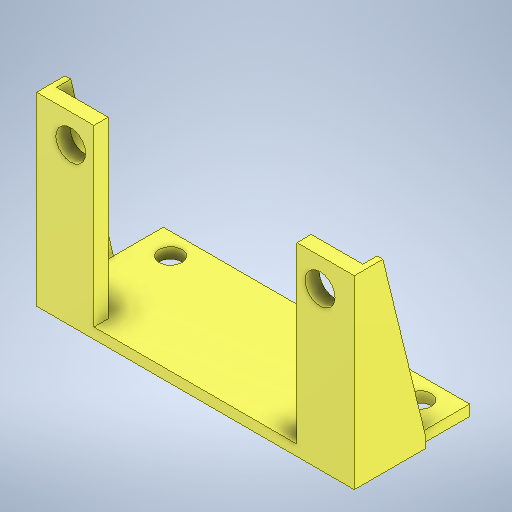
# Autodesk Inventor part: 28BYJ-48_Braket3
Saved by Autodesk Inventor 2025.3 (Build 293356030, 356C)
## iProperties
Created: 2025-07-13
Part Number: 28BYJ-48_Braket3
Material: 一般
Document SubType Name: Modeling
Designer: daisuke
Density: 1 g/cm^3
Appearance: 滑らか - 黄
Author: daisuke
Autodesk Inventor part; units mm, degrees
ref_plane "YZ Plane" through (0, 0, 0) normal (1, 0, 0) x (0, 1, 0)
ref_plane "XZ Plane" through (0, 0, 0) normal (0, 1, 0) x (-1, 0, 0)
ref_plane "XY Plane" through (0, 0, 0) normal (0, 0, 1) x (1, 0, 0)
sketch "スケッチ1" plane through (0, 0, 0) normal (0, 0, 1) x (1, 0, 0)
  line L0 (0, 0) -> (0, 23.3181) construction
  line L1 (-22.6457, 22) -> (22.6457, 22) construction
  line L2 (-20.3832, 1.5) -> (20.3832, 1.5) construction
  circle A0 centre (0, 22) radius 14 construction
  line L3 (-22.6457, 14) -> (22.6457, 14) construction
  circle A1 centre (-17.5, 22) radius 2.1
  circle A2 centre (17.5, 22) radius 2.1
  line L4 (-21.5, 26) -> (-21.5, 0)
  line L5 (-21.5, 0) -> (-14.25, 0)
  line L6 (-14.25, 0) -> (-14.25, 26)
  line L7 (21.5, 26) -> (21.5, 0)
  line L8 (21.5, 0) -> (14.25, 0)
  line L9 (14.25, 0) -> (14.25, 26)
  line L10 (-14.25, 26) -> (-21.5, 26)
  line L11 (14.25, 26) -> (21.5, 26)
  line L12 (21.5, 1.5) -> (-21.5, 1.5)
  line L13 (-21.5, 1.5) -> (-21.5, 0)
  line L14 (-21.5, 0) -> (21.5, 0)
  line L15 (21.5, 0) -> (21.5, 1.5)
  point P0 (0, 1.5)
  point P1 (0, 14)
  point P2 (14.25, 1.5)
  point P3 (-14.25, 1.5)
  point P4 (0, 0)
  dimension "d0" = 28
  dimension "d1" = 1.5
  dimension "d2" = 8
  dimension "d3" = 4.2
  dimension "d4" = 35
  dimension "d29" = 3.25
  dimension "d30" = 3.25
  dimension "d31" = 4
  dimension "d32" = 4
  dimension "d46" = 22
  dimension "d47" = 4
  constraints: 32 end point, 8 point on line, 5 equal length, 5 horizontal, 4 midpoint, 3 centre point, 3 vertical, 2 perpendicular, 1 coincident, 1 collinear, 1 equal radius, 1 horizontal alignment, 1 symmetric about line
  measures "d0" diameter of A0
  measures "d1" distance from line of L2 L0.start
  measures "d2" distance between parallel lines of L3 L1
  measures "d3" diameter of A1
  measures "d4" distance of A2.centre A1.centre
  measures "d29" distance from line of L6 A1.centre
  measures "d30" distance from line of L9 A2.centre
  measures "d31" distance from line of L4 A1.centre
  measures "d32" distance from line of L7 A2.centre
  measures "d46" distance from line of point (0, 0) L1
  measures "d47" distance between parallel lines of L10 L1
extrude "前" add sketch "スケッチ1" along normal blind 2
extrude "底" add sketch "スケッチ1" against normal blind 15 contours L12 L6 L5 L4 | L12 L9 L14 L6 | L12 L7 L8 L9
sketch "スケッチ5" plane through (-14.25, 1.5, 2) normal (0, 1, 0) x (1, 0, 0)
  line L0 (14.25, -6.214) -> (14.25, 25.3742) construction
  line L1 (28.5, 0) -> (0, 0) construction
  point P0 (14.25, 2)
  point P1 (-3.25, 14)
  point P2 (31.75, 14)
  dimension "d33" = 35
  dimension "d34" = 14
  constraints: 2 end point, 1 point on line, 1 symmetric about line, 1 vertical
  measures "d33" distance of point (31.75, 14) point (-3.25, 14)
  measures "d34" distance from line of L1 point (-3.25, 14)
hole "穴2" at (-17.5, 1.5, -12) at (17.5, 1.5, -12) direction (0, -1, 0) diameter 3.2 end through all
sketch "スケッチ6" plane through (21.5, 1.5, 0) normal (1, 0, 0) x (0, 0, -1)
  line L0 (2, 24.5) -> (-2, 24.5)
  line L1 (-2, 24.5) -> (-2, 0) projected
  line L2 (-2, 24.5) -> (-2, -1.5)
  line L3 (-2, -1.5) -> (8, -1.5)
  line L4 (8, -1.5) -> (8, 0)
  line L5 (8, 0) -> (2, 24.5)
  point P0 (0, -1.5)
  point P1 (15, 0)
  dimension "d42" = 4
  dimension "d43" = 10
  constraints: 10 end point, 4 perpendicular, 1 horizontal alignment
  measures "d42" distance of L0.start L0.end
  measures "d43" distance of L2.end L3.end
extrude "押し出し5" add sketch "スケッチ6" along normal blind 0.8
mirror "ミラー3" about plane through (0, 0, 0) normal (1, 0, 0) of "押し出し5"
equation "\"d30\" = d29"
equation "\"d32\" = d31"
